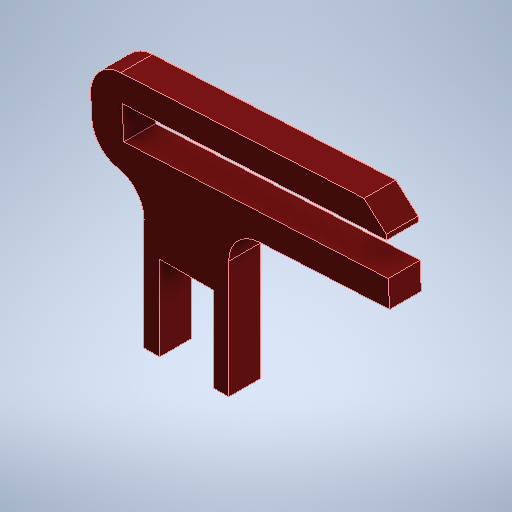
# Autodesk Inventor part: Path Plate Connector
Saved by Autodesk Inventor 2025.4 (Build 294407000, 407)
## iProperties
Created: 2026-05-18
Part Number: Path Plate Connector
Material: Generic
Document SubType Name: Sheet Metal
Designer: lenovo
Density: 1 g/cm^3
Sheet Metal Rule: Default_mm
Appearance: Default(1)
Author: lenovo
Autodesk Inventor part; units mm, degrees
ref_plane "YZ Plane" through (0, 0, 0) normal (1, 0, 0) x (0, 1, 0)
ref_plane "XZ Plane" through (0, 0, 0) normal (0, 1, 0) x (-1, 0, 0)
ref_plane "XY Plane" through (0, 0, 0) normal (0, 0, 1) x (1, 0, 0)
sketch "Sketch1" plane through (0, 0, 0) normal (0, 0, 1) x (1, 0, 0)
  line L0 (-4, -7) -> (4, -7)
  line L1 (4, -7) -> (4, 7)
  line L2 (4, 7) -> (-4, 7)
  line L3 (-4, 7) -> (-4, -7)
  line L4 (-4, -7) -> (4, 7) construction
  line L5 (4, -7) -> (-4, 7) construction
  line L6 (19.1902, 7.7382) -> (18.7715, 15.7272)
  line L7 (18.7715, 15.7272) -> (-9.1902, 14.2618)
  line L8 (-9.1902, 14.2618) -> (-8.7715, 6.2728)
  line L9 (-8.7715, 6.2728) -> (19.1902, 7.7382)
  line L10 (19.1902, 7.7382) -> (-9.1902, 14.2618) construction
  line L11 (18.7715, 15.7272) -> (-8.7715, 6.2728) construction
  line L12 (19.0606, 10.2098) -> (18.901, 13.2556)
  line L13 (18.901, 13.2556) -> (-6.0647, 11.9472)
  line L14 (-6.0647, 11.9472) -> (-5.9051, 8.9014)
  line L15 (-5.9051, 8.9014) -> (19.0606, 10.2098)
  line L16 (-8.9808, 10.2673) -> (18.9808, 11.7327)
  line L17 (-2.525, -7) -> (2.525, -7)
  line L18 (2.525, -7) -> (2.525, 1)
  line L19 (2.525, 1) -> (-2.525, 1)
  line L20 (-2.525, 1) -> (-2.525, -7)
  point P0 (0, 0)
  point P1 (0, 0)
  point P2 (5, 11)
  point P3 (5, 11)
  point P4 (5, 11)
  point P5 (0, 1)
  point P6 (0, -7)
  point P7 (-4, 6.5228)
  point P8 (4, 6.9421)
  point P9 (19.0606, 10.2098)
  point P10 (18.901, 13.2556)
  dimension "d19" = 8
  dimension "d20" = 14
  dimension "d21" = 5
  dimension "d22" = 3
  dimension "d23" = 4
  dimension "d24" = 8
  dimension "d25" = 28
  dimension "d27" = 3.05
  dimension "d29" = 25
  dimension "d30" = 5.05
  dimension "d31" = 8
  measures "d19" distance of L2.end L1.end
  measures "d20" distance of L1.end L0.end
  measures "d21" horizontal distance of point (0, 0) point (5, 11)
  measures "d22" angle of L7 L2
  measures "d23" distance from line of L2 point (5, 11)
  measures "d24" distance between parallel lines of L7 L9
  measures "d25" distance between parallel lines of L6 L8
  measures "d27" distance between parallel lines of L13 L15
  measures "d29" distance between parallel lines of L12 L14
  measures "d30" distance of L18.end L19.end
  measures "d31" distance of L17.end L18.end
extrude "Plate1" add sketch "Sketch1" along normal blind 3 contours L3 L9 L1 L0 L18 L19 L20 | L9 L8 L16 L14 L15 L6 L1 L2 L3 | L3 L2 L1 L9 | L8 L7 L6 L13 L14 L16
chamfer "Corner Chamfer1" distance 2 angle 45 1 edges at (18.7715, 15.7272, 1.5)
fillet "Corner Round2" radius 3 4 edges at (4, 6.9421, 1.5) (-8.7715, 6.2728, 1.5) (-4, 6.5228, 1.5) (-9.1902, 14.2618, 1.5)
equation "\"d14\" = Thickness"
equation "\"BendRadius\" = Thickness"
equation "\"BendReliefWidth\" = Thickness"
equation "\"BendReliefDepth\" = 0.5 * Thickness"
equation "\"CornerReliefSize\" = 4 * Thickness"
equation "\"MinimumRemnant\" = 2 * Thickness"
equation "\"TransitionRadius\" = BendRadius"
equation "\"JacobiRadiusSize\" = BendRadius"
equation "\"GapSize\" = Thickness"
equation "\"Thickness\" = 3"
body "Solid1"
